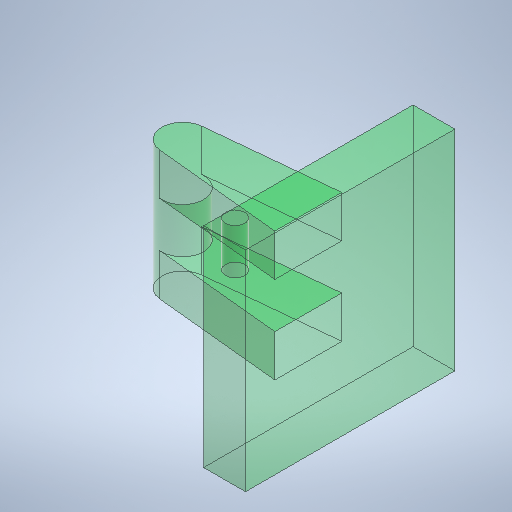
# Autodesk Inventor part: Pieza2PrimerEslabon
Saved by Autodesk Inventor 2025.2 (Build 292293000, 293)
## iProperties
Created: 2025-03-31
Part Number: Pieza2PrimerEslabon
Material: Cristal
Document SubType Name: Modeling
Designer: braug
Density: 2.18 g/cm^3
Appearance: Claro
Author: braug
Autodesk Inventor part; units mm, degrees
ref_plane "YZ Plane" through (0, 0, 0) normal (1, 0, 0) x (0, 1, 0)
ref_plane "XZ Plane" through (0, 0, 0) normal (0, 1, 0) x (-1, 0, 0)
ref_plane "XY Plane" through (0, 0, 0) normal (0, 0, 1) x (1, 0, 0)
sketch "Boceto1" plane through (0, 0, 0) normal (0, 1, 0) x (-1, 0, 0)
  circle A0 centre (0, 0) radius 5
  circle A1 centre (-12.5, 0) radius 2.3
  dimension "d0" = 10
  dimension "d1" = 4.6
  constraints: 2 centre point
  measures "d0" diameter of A0
  measures "d1" diameter of A1
extrude "Extrusión1" add sketch "Boceto1" along normal blind 10.8
sketch "Boceto2" plane through (0, 10.8, 0) normal (0, 1, 0) x (1, 0, 0)
  circle A0 centre (0, 0) radius 5
  line L0 (30, 0) -> (30, -10)
  line L1 (-0.4927, -4.9757) -> (30, -7.9951)
  line L2 (30, 0) -> (30, 10)
  line L3 (-0.4927, 4.9757) -> (30, 7.9951)
  constraints: 8 end point, 2 point on line, 1 centre point
extrude "Extrusión2" add sketch "Boceto2" along normal blind 10
sketch "Boceto3" plane through (0, 0, 0) normal (0, -1, 0) x (1, 0, 0)
  line L0 (30, -7.9951) -> (-0.4927, -4.9757) projected
  line L1 (30, 7.9951) -> (30, -7.9951) projected
  line L2 (-0.4927, 4.9757) -> (30, 7.9951) projected
  circle A0 centre (0, 0) radius 5 projected
extrude "Extrusión3" add sketch "Boceto3" along normal blind 10
sketch "Boceto4" plane through (30, 10.8, 7.9951) normal (1, 0, 0) x (0, 0, -1)
  line L0 (0, 0) -> (15.9902, 0) projected
  line L1 (7.9951, 0) -> (7.9951, -10.8) construction
  line L2 (32.9951, 19.6) -> (-17.0049, 19.6)
  line L3 (-17.0049, 19.6) -> (-17.0049, -30.4)
  line L4 (-17.0049, -30.4) -> (32.9951, -30.4)
  line L5 (32.9951, -30.4) -> (32.9951, 19.6)
  line L6 (32.9951, 19.6) -> (-17.0049, -30.4) construction
  line L7 (-17.0049, 19.6) -> (32.9951, -30.4) construction
  point P0 (7.9951, -5.4)
  dimension "d10" = 50
  dimension "d11" = 50
  constraints: 14 end point, 4 midpoint, 2 parallel, 1 horizontal, 1 perpendicular, 1 vertical
  measures "d10" distance of L4.end L3.end
  measures "d11" distance of L3.end L2.end
extrude "Extrusión4" add sketch "Boceto4" along normal blind 10
